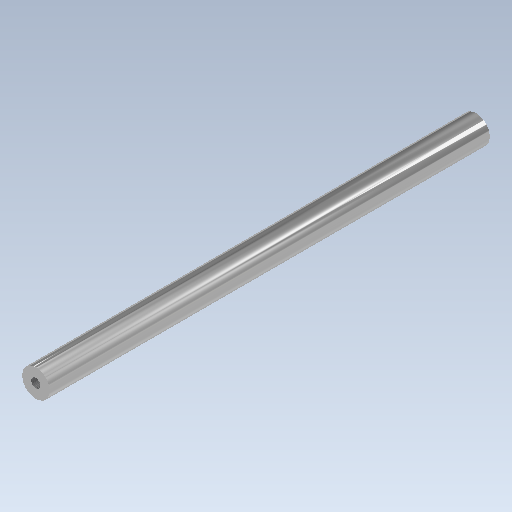
# Autodesk Inventor part: ADSK-MH-10018
Saved by Autodesk Inventor 2020.2 (Build 242310000, 310)
## iProperties
Created: 2008-03-10
Part Number: ADSK-MH-10018
Document SubType Name: Modeling
Designer: R.O'mahony
Density: 7.86 g/cm^3
Mass: 274.496 g
Surface Area: 466.908 cm^2
Volume: 274.496 cm^3
Material: Steel, Mild
Description: Support Bar Long.ipt
Appearance: Chrome - Polished
Engineer: Demir Ali
Checked By: Demir Ali
Company: Autodesk Ltd
Author: R.O'mahony
Keywords: Roller Conveyor
Revision Number: A
Autodesk Inventor part; units mm, degrees
ref_plane "YZ Plane" through (0, 0, 0) normal (1, 0, 0) x (0, 1, 0)
ref_plane "XZ Plane" through (0, 0, 0) normal (0, 1, 0) x (-1, 0, 0)
ref_plane "XY Plane" through (0, 0, 0) normal (0, 0, 1) x (1, 0, 0)
sketch "Sketch1" plane through (0, 0, 0) normal (0, 0, 1) x (1, 0, 0)
  circle A0 centre (0, 0) radius 12.5
  dimension "d0" = 25
  constraints: 1 centre point, 1 coincident
  measures "d0" diameter of A0
extrude "Extrusion1" add sketch "Sketch1" along normal mid plane 400
sketch "Sketch2" plane through (0, 0, 200) normal (0, 0, 1) x (1, 0, 0)
  circle A0 centre (0, 0) radius 12.5 projected
  constraints: 1 coincident
hole "Hole1" at (0, 0, 200) direction (0, 0, -1) diameter 8.376 depth 25 tip angle 118 thread size "M10x1.5" class "6H" standard "ISO Metric profile"
mirror "Mirror1" about plane through (0, 0, 0) normal (0, 0, 1) of "Hole1"
body "Solid1"
